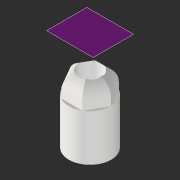
# Autodesk Inventor part: stick
Saved by Autodesk Inventor 2020.3 (Build 243373010, 373A)
## iProperties
Created: 2021-01-25
Part Number: stick
Material: Generic
Document SubType Name: Modeling
Designer: Melvin Strobl
Density: 1 g/cm^3
Appearance: Default
Author: Melvin Strobl
Autodesk Inventor part; units mm, degrees
ref_plane "YZ Plane" through (0, 0, 0) normal (1, 0, 0) x (0, 1, 0)
ref_plane "XZ Plane" through (0, 0, 0) normal (0, 1, 0) x (-1, 0, 0)
ref_plane "XY Plane" through (0, 0, 0) normal (0, 0, 1) x (1, 0, 0)
sketch "Sketch1" plane through (0, 0, 0) normal (0, 1, 0) x (-1, 0, 0)
  line L0 (4.5611, 0) -> (2.2805, -3.95)
  line L1 (2.2805, -3.95) -> (-2.2805, -3.95)
  line L2 (-2.2805, -3.95) -> (-4.5611, 0)
  line L3 (-4.5611, 0) -> (-2.2805, 3.95)
  line L4 (-2.2805, 3.95) -> (2.2805, 3.95)
  line L5 (2.2805, 3.95) -> (4.5611, 0)
  circle A0 centre (0, 0) radius 1.5
  circle A1 centre (0, 0) radius 2.45
  circle A2 centre (0, 0) radius 4.5611
  point P0 (-2.2805, -3.95)
  point P1 (-2.2805, -3.95)
  dimension "d0" = 7.9
  dimension "d5" = 3
  dimension "d6" = 4.9
  constraints: 12 end point, 3 coincident, 2 centre point, 16 other
  measures "d0" distance between parallel lines of L1 L4
  measures "d5" diameter of A0
  measures "d6" diameter of A1
extrude "Extrusion1" add sketch "Sketch1" along normal blind 15 contours L0 L1 L2 L3 L4 L5 | A0 | A1
fillet "Fillet1" radius 3.5 6 edges at (3.4208, 15, 1.975) (0, 15, 3.95) (-3.4208, 15, 1.975) (-3.4208, 15, -1.975) (0, 15, -3.95) (3.4208, 15, -1.975)
extrude "Extrusion2" cut sketch "Sketch1" along normal blind 2.5 contours A1
extrude "Extrusion3" cut sketch "Sketch1" along normal blind 27 contours A0
ref_plane "Work Plane1" through (0, 21.5, 0) normal (0, -1, 0) x (1, 0, 0)
extrude "Extrusion4" cut sketch "Sketch1" against normal blind 17.5 from surface at 21.5 contours A1
fillet "Fillet2" radius 1.4 1 edges at (2.45, 2.5, 0)
fillet "Fillet3" radius 0.3 1 edges at (2.45, 4, 0)
extrude "Extrusion5" add sketch "Sketch1" along normal blind 10 contours A2 L0 | L5 A2 | A2 L1 | L4 A2 | A2 L2 | L3 A2
body "Solid1"
